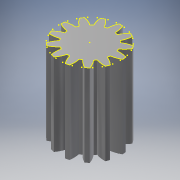
# Autodesk Inventor part: 平歯車1
Saved by Autodesk Inventor 2018.3 (Build 223284000, 284)
## iProperties
Created: 2019-04-14
Part Number: 平歯車1
Material: Steel
Document SubType Name: Modeling
Designer: shun2
Categories: <?xml version="1.0" encoding="UTF-16"?> <MemberInstance><Categories><FamilyTemplate><FamilyTemplateParameter ValueType="xs:double" Id="1" ObjectReferenceKey="da_z" ObjectType="kUserParameterObject"/><FamilyTemplateParameter ValueType="xs:double" Id="2" ObjectReferenceKey="da_b" ObjectType="kUserParameterObject"/><FamilyTemplateParameter ValueType="xs:double" Id="3" ObjectReferenceKey="da_beta" ObjectType="kUserParameterObject"/><FamilyTemplateParameter ValueType="xs:double" Id="4" ObjectReferenceKey="da_da" ObjectType="kUserParameterObject"/><FamilyTemplateParameter ValueType="xs:double" Id="5" ObjectReferenceKey="da_aw" ObjectType="kUserParameterObject"/><FamilyTemplateParameter ValueType="xs:string" Id="6" ObjectReferenceKey="EAIAABAAAACIAQAAAAAAAIAAAAAAAAAA" ObjectType="83910656" SubObjectId="SurfaceGeometry"/></FamilyTemplate><ParamToTemplateMap><ParamToTemplate CategoryParameter="//CategoryParameter[@InternalName='046C89C9-8512-4d59-83FE-43B91F4F132A']" TemplateParameter="1"/><ParamToTemplate CategoryParameter="//CategoryParameter[@InternalName='2552DF32-E462-4b46-AEBF-C6C7768E72AC']" TemplateParameter="2"/><ParamToTemplate CategoryParameter="//CategoryParameter[@InternalName='C9EE641D-15FC-4fae-A226-E94C4372FDD7']" TemplateParameter="3"/><ParamToTemplate><ParamToTemplate CategoryParameter="//CategoryParameter[@InternalName='00B6519A-459B-49c7-AD84-2E56D39A5744']" ConstantValue="-0.000000"/></ParamToTemplate><ParamToTemplate><ParamToTemplate CategoryParameter="//CategoryParameter[@InternalName='04B31F0E-C7A6-4894-AA32-9629BEFACF47']" ConstantValue="1.000000"/></ParamToTemplate><ParamToTemplate><ParamToTemplate CategoryParameter="//CategoryParameter[@InternalName='43CBEC2E-7847-49e7-A936-2F7889FCB2D9']" ConstantValue="0.250000"/></ParamToTemplate><ParamToTemplate><ParamToTemplate CategoryParameter="//CategoryParameter[@InternalName='B1EFC894-105D-4ebd-86BF-FA20ED196853']" ConstantValue="0.333500"/></ParamToTemplate><ParamToTemplate><ParamToTemplate CategoryParameter="//CategoryParameter[@InternalName='51175063-3D10-4879-93E8-6246FE8B403D']" ConstantValue="2060000000.000000"/></ParamToTemplate><ParamToTemplate><ParamToTemplate CategoryParameter="//CategoryParameter[@InternalName='A3A52E27-4454-46a9-B0BD-C932399B70AF']" ConstantValue="0.300000"/></ParamToTemplate><ParamToTemplate><ParamToTemplate CategoryParameter="//CategoryParameter[@InternalName='91B76062-C214-41d9-B1B9-14D2AB99603D']" ConstantValue="0.100000"/></ParamToTemplate><ParamToTemplate><ParamToTemplate CategoryParameter="//CategoryParameter[@InternalName='374E806E-8B8A-4dda-A9AA-1039D6500AD2']" ConstantValue="10.000000"/></ParamToTemplate><ParamToTemplate><ParamToTemplate CategoryParameter="//CategoryParameter[@InternalName='2D373A89-B862-43d6-8D0B-0CBF12AB9F6C']" ConstantValue="0.253073"/></ParamToTemplate><ParamToTemplate CategoryParameter="//CategoryParameter[@InternalName='37777632-D6A2-4fac-9D53-DB8ACD95C989']" TemplateParameter="4"/><ParamToTemplate CategoryParameter="//CategoryParameter[@InternalName='FD1017F1-B727-4f7e-9707-0F86F1FF9423']" TemplateParameter="5"/><ParamToTemplate><ParamToTemplate CategoryParameter="//CategoryParameter[@InternalName='9E1B4470-B2D3-4ff1-B813-535BB4CDF51A']" ConstantValue="3520000.000000"/></ParamToTemplate><ParamToTemplate><ParamToTemplate CategoryParameter="//CategoryParameter[@InternalName='F8452263-BFF6-458c-9FB1-07C4B99E95CD']" ConstantValue="11400000.000000"/></ParamToTemplate><ParamToTemplate><ParamToTemplate CategoryParameter="//CategoryParameter[@InternalName='3E3BB259-FD49-497f-8171-6EBC954A3479']" ConstantValue="2.000000"/></ParamToTemplate><ParamToTemplate CategoryParameter="//CategoryParameter[@InternalName='27C3BAF2-7550-4e4b-AE2C-0DB134B7D9B7']" TemplateParameter="6"/></ParamToTemplateMap><Category DisplayName="Gear" InternalName="DC85795E-93AB-48d5-8EEE-5A27447B64BD" Mnemonic="Gear"><CategoryParameter DisplayName="z" InternalName="046C89C9-8512-4d59-83FE-43B91F4F132A" Mnemonic="z"/><CategoryParameter DisplayName="b" InternalName="2552DF32-E462-4b46-AEBF-C6C7768E72AC" Mnemonic="b"/><CategoryParameter DisplayName="||b|" InternalName="C9EE641D-15FC-4fae-A226-E94C4372FDD7" Mnemonic="beta"/><CategoryParameter DisplayName="x" InternalName="00B6519A-459B-49c7-AD84-2E56D39A5744" Mnemonic="x"/><CategoryParameter DisplayName="a*" InternalName="04B31F0E-C7A6-4894-AA32-9629BEFACF47" Mnemonic="a"/><CategoryParameter DisplayName="c*" InternalName="43CBEC2E-7847-49e7-A936-2F7889FCB2D9" Mnemonic="c"/><CategoryParameter DisplayName="r|.f|*" InternalName="B1EFC894-105D-4ebd-86BF-FA20ED196853" Mnemonic="rf"/><CategoryParameter DisplayName="E" InternalName="51175063-3D10-4879-93E8-6246FE8B403D" Mnemonic="E"/><CategoryParameter DisplayName="||m|" InternalName="A3A52E27-4454-46a9-B0BD-C932399B70AF" Mnemonic="mi"/><Category DisplayName="SpurGear" InternalName="26C5A22E-A91E-4dfd-A3B3-23CCAFAE1764" Mnemonic="SpurGear"><CategoryParameter DisplayName="m" InternalName="91B76062-C214-41d9-B1B9-14D2AB99603D" Mnemonic="m"/><CategoryParameter DisplayName="P" InternalName="374E806E-8B8A-4dda-A9AA-1039D6500AD2" Mnemonic="PP"/><CategoryParameter DisplayName="||a|" InternalName="2D373A89-B862-43d6-8D0B-0CBF12AB9F6C" Mnemonic="alpha"/><CategoryParameter DisplayName="d|.a|" InternalName="37777632-D6A2-4fac-9D53-DB8ACD95C989" Mnemonic="da"/><CategoryParameter DisplayName="a|.w|" InternalName="FD1017F1-B727-4f7e-9707-0F86F1FF9423" Mnemonic="aw"/><CategoryParameter DisplayName="||s||.Flim|" InternalName="9E1B4470-B2D3-4ff1-B813-535BB4CDF51A" Mnemonic="sFlim"/><CategoryParameter DisplayName="||s||.Hlim|" InternalName="F8452263-BFF6-458c-9FB1-07C4B99E95CD" Mnemonic="sHlim"/><CategoryParameter DisplayName="種類" InternalName="3E3BB259-FD49-497f-8171-6EBC954A3479" Mnemonic="type"/><CategoryParameter DisplayName="PitchDiameter" InternalName="27C3BAF2-7550-4e4b-AE2C-0DB134B7D9B7" Mnemonic="IDS_PITCHDIAM"/></Category></Category></Categories></MemberInstance>
Density: 1 g/cm^3
Appearance: Steel
CustomPartVersion: 1
Author: shun2
Autodesk Inventor part; units mm, degrees
sketch "Sketch1" plane through (0, 0, 0) normal (0, 0, 1) x (1, 0, 0)
  circle A0 centre (0, 0) radius 7.5
  dimension "d0" = 15
  constraints: 1 centre point
  measures "d0" diameter of A0
extrude "Extrusion1" add sketch "Sketch1" along normal blind 20
ref_plane "Work Plane2" through (0, 0, 10) normal (0, 0, 1) x (1, 0, 0)
sketch "Sketch2" plane through (0, 0, 0) normal (0, 0, -1) x (-1, 0, 0)
  circle A0 centre (0, 0) radius 7.5 projected
  circle A1 centre (0, 0) radius 6.5
  dimension "d3" = 13
  constraints: 1 centre point, 1 coincident
  measures "d3" diameter of A1
surface extrude "ピッチ円直径" sketch "Sketch2" against normal through all shown no curves A1
ref_plane "Work Plane8" through (0, 0, 0) normal (0.9709418, 0.2393157, 0) x (0, 0, 1)
ref_plane "Work Plane9" through (0, 0, 0) normal (1, 0, 0) x (0, 1, 0)
spur gear teeth "平歯車" teeth 13 pitch diameter 13 tip diameter 15 root diameter 10.5 face width 20 start plane through (0, 0, 0) normal (0, 0, -1) x (-1, 0, 0)
sketch "スケッチ3" plane through (0, 0, 20) normal (0, 0, 1) x (1, 0, 0)
  arc A0 (-3.88, 6.4184) -> (-3.2378, 4.1327) centre (2.5862, 7.0023) ccw projected
  arc A1 (-3.2378, 4.1327) -> (-3.7123, 3.7123) centre (0, 0) ccw projected
  arc A2 (-3.7123, 3.7123) -> (-5.9039, 4.6254) centre (-7.263, -1.7233) ccw projected
  arc A3 (-5.9039, 4.6254) -> (-6.4184, 3.88) centre (0, 0) ccw projected
  arc A4 (-6.4184, 3.88) -> (-4.7875, 2.1547) centre (-0.9641, 7.4021) ccw projected
  arc A5 (-4.7875, 2.1547) -> (-5.0123, 1.5619) centre (0, 0) ccw projected
  arc A6 (-5.0123, 1.5619) -> (-7.3771, 1.3519) centre (-5.6302, -4.9012) ccw projected
  arc A7 (-7.3771, 1.3519) -> (-7.4863, 0.4528) centre (0, 0) ccw projected
  arc A8 (-7.4863, 0.4528) -> (-5.2404, -0.317) centre (-4.2936, 6.1062) ccw projected
  arc A9 (-5.2404, -0.317) -> (-5.164, -0.9463) centre (0, 0) ccw projected
  arc A10 (-5.164, -0.9463) -> (-7.1604, -2.2313) centre (-2.7076, -6.9563) ccw projected
  arc A11 (-7.1604, -2.2313) -> (-6.8392, -3.0781) centre (0, 0) ccw projected
  arc A12 (-6.8392, -3.0781) -> (-4.4929, -2.716) centre (-6.6395, 3.4114) ccw projected
  arc A13 (-4.4929, -2.716) -> (-4.1327, -3.2378) centre (0, 0) ccw projected
  arc A14 (-4.1327, -3.2378) -> (-5.3033, -5.3033) centre (0.8353, -7.4178) ccw projected
  arc A15 (-5.3033, -5.3033) -> (-4.6254, -5.9039) centre (0, 0) ccw projected
  arc A16 (-4.6254, -5.9039) -> (-2.716, -4.4929) centre (-7.4644, -0.0649) ccw projected
  arc A17 (-2.716, -4.4929) -> (-2.1547, -4.7875) centre (0, 0) ccw projected
  arc A18 (-2.1547, -4.7875) -> (-2.2313, -7.1604) centre (4.1868, -6.1799) ccw projected
  arc A19 (-2.2313, -7.1604) -> (-1.3519, -7.3771) centre (0, 0) ccw projected
  arc A20 (-1.3519, -7.3771) -> (-0.317, -5.2404) centre (-6.5792, -3.5263) ccw projected
  arc A21 (-0.317, -5.2404) -> (0.317, -5.2404) centre (0, 0) ccw projected
  arc A22 (0.317, -5.2404) -> (1.3519, -7.3771) centre (6.5792, -3.5263) ccw projected
  arc A23 (1.3519, -7.3771) -> (2.2313, -7.1604) centre (0, 0) ccw projected
  arc A24 (2.2313, -7.1604) -> (2.1547, -4.7875) centre (-4.1868, -6.1799) ccw projected
  arc A25 (2.1547, -4.7875) -> (2.716, -4.4929) centre (0, 0) ccw projected
  arc A26 (2.716, -4.4929) -> (4.6254, -5.9039) centre (7.4644, -0.0649) ccw projected
  arc A27 (4.6254, -5.9039) -> (5.3033, -5.3033) centre (0, 0) ccw projected
  arc A28 (5.3033, -5.3033) -> (4.1327, -3.2378) centre (-0.8353, -7.4178) ccw projected
  arc A29 (4.1327, -3.2378) -> (4.4929, -2.716) centre (0, 0) ccw projected
  arc A30 (4.4929, -2.716) -> (6.8392, -3.0781) centre (6.6395, 3.4114) ccw projected
  arc A31 (6.8392, -3.0781) -> (7.1604, -2.2313) centre (0, 0) ccw projected
  arc A32 (7.1604, -2.2313) -> (5.164, -0.9463) centre (2.7076, -6.9563) ccw projected
  arc A33 (5.164, -0.9463) -> (5.2404, -0.317) centre (0, 0) ccw projected
  arc A34 (5.2404, -0.317) -> (7.4863, 0.4528) centre (4.2936, 6.1062) ccw projected
  arc A35 (7.4863, 0.4528) -> (7.3771, 1.3519) centre (0, 0) ccw projected
  arc A36 (7.3771, 1.3519) -> (5.0123, 1.5619) centre (5.6302, -4.9012) ccw projected
  arc A37 (5.0123, 1.5619) -> (4.7875, 2.1547) centre (0, 0) ccw projected
  arc A38 (4.7875, 2.1547) -> (6.4184, 3.88) centre (0.9641, 7.4021) ccw projected
  arc A39 (6.4184, 3.88) -> (5.9039, 4.6254) centre (0, 0) ccw projected
  arc A40 (5.9039, 4.6254) -> (3.7123, 3.7123) centre (7.263, -1.7233) ccw projected
  arc A41 (3.7123, 3.7123) -> (3.2378, 4.1327) centre (0, 0) ccw projected
  arc A42 (3.2378, 4.1327) -> (3.88, 6.4184) centre (-2.5862, 7.0023) ccw projected
  arc A43 (3.88, 6.4184) -> (3.0781, 6.8392) centre (0, 0) ccw projected
  arc A44 (3.0781, 6.8392) -> (1.5619, 5.0123) centre (7.2319, 1.8493) ccw projected
  arc A45 (1.5619, 5.0123) -> (0.9463, 5.164) centre (0, 0) ccw projected
  arc A46 (0.9463, 5.164) -> (0.4528, 7.4863) centre (-5.5441, 4.9983) ccw projected
  arc A47 (0.4528, 7.4863) -> (-0.4528, 7.4863) centre (0, 0) ccw projected
  arc A48 (-0.4528, 7.4863) -> (-0.9463, 5.164) centre (5.5441, 4.9983) ccw projected
  arc A49 (-0.9463, 5.164) -> (-1.5619, 5.0123) centre (0, 0) ccw projected
  arc A50 (-1.5619, 5.0123) -> (-3.0781, 6.8392) centre (-7.2319, 1.8493) ccw projected
  arc A51 (-3.0781, 6.8392) -> (-3.88, 6.4184) centre (0, 0) ccw projected
equation "\"d0\" = da_da"
equation "\"d1\" = da_b"
equation "\"d3\" = da_dw"
equation "\"da_da\" = 15"
equation "\"da_b\" = 20"
equation "\"da_dw\" = 13"
body "Solid1"
body "Srf1"
